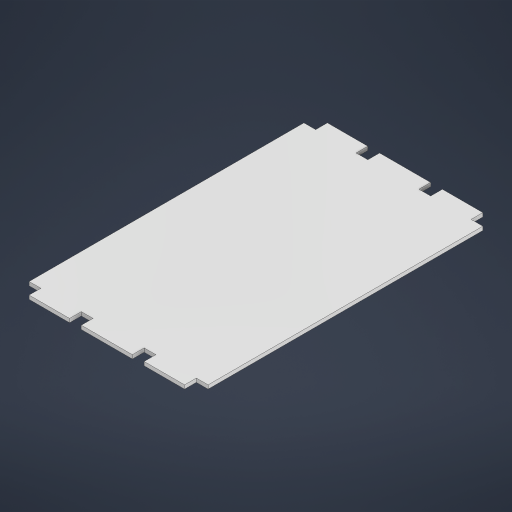
# Autodesk Inventor part: Shee
Saved by Autodesk Inventor 2024.3 (Build 283343000, 343)
## iProperties
Created: 2024-06-13
Part Number: Shee
Material: Generic
Document SubType Name: Modeling
Designer: braed
Density: 1 g/cm^3
Appearance: Default
Author: braed
Autodesk Inventor part; units mm, degrees
ref_plane "YZ Plane" through (0, 0, 0) normal (1, 0, 0) x (0, 1, 0)
ref_plane "XZ Plane" through (0, 0, 0) normal (0, 1, 0) x (-1, 0, 0)
ref_plane "XY Plane" through (0, 0, 0) normal (0, 0, 1) x (1, 0, 0)
sketch "Sketch1" plane through (0, 0, 0) normal (0, 0, 1) x (1, 0, 0)
  line L0 (0, 0) -> (304.8, 0)
  line L1 (304.8, 0) -> (304.8, 6.35)
  line L2 (304.8, 6.35) -> (0, 6.35)
  line L3 (0, 6.35) -> (0, 0)
  dimension "d0" = 304.8
  dimension "d1" = 6.35
  constraints: 8 end point, 2 parallel, 1 horizontal, 1 perpendicular
  measures "d0" distance of L2.end L1.end
  measures "d1" distance of L1.end L0.end
extrude "Extrusion1" add sketch "Sketch1" along normal blind 508
sketch "Sketch2" plane through (0, 6.35, 0) normal (0, 1, 0) x (1, 0, 0)
  line L0 (304.8, 0) -> (0, 0) construction
  line L1 (152.4, 0) -> (152.4, -508) construction
  line L2 (304.8, -508) -> (0, -508) construction
  line L3 (0, 0) -> (0, -508) construction
  line L4 (0, -254) -> (304.8, -254) construction
  line L5 (304.8, 0) -> (304.8, -508) construction
  line L6 (0, 0) -> (0, -20)
  line L7 (0, -20) -> (20, -20) construction
  line L8 (20, -20) -> (0, -20)
  line L9 (0, -20) -> (0, 0)
  line L10 (0, 0) -> (20, 0)
  line L11 (20, 0) -> (20, -20)
  line L12 (304.8, 0) -> (304.8, -20)
  line L13 (304.8, -20) -> (284.8, -20) construction
  line L14 (284.8, -20) -> (304.8, -20)
  line L15 (304.8, -20) -> (304.8, 0)
  line L16 (304.8, 0) -> (284.8, 0)
  line L17 (284.8, 0) -> (284.8, -20)
  line L18 (304.8, -508) -> (0, -508) construction
  line L19 (0, -508) -> (0, -488)
  line L20 (0, -488) -> (20, -488) construction
  line L21 (20, -488) -> (0, -488)
  line L22 (0, -488) -> (0, -508)
  line L23 (0, -508) -> (20, -508)
  line L24 (20, -508) -> (20, -488)
  line L25 (304.8, -508) -> (304.8, -488)
  line L26 (304.8, -488) -> (284.8, -488) construction
  line L27 (284.8, -488) -> (304.8, -488)
  line L28 (304.8, -488) -> (304.8, -508)
  line L29 (304.8, -508) -> (284.8, -508)
  line L30 (284.8, -508) -> (284.8, -488)
  dimension "d4" = 20
  dimension "d5" = 20
  constraints: 54 end point, 12 symmetric about line, 4 midpoint, 2 parallel, 2 perpendicular, 1 horizontal, 1 point on line
  measures "d4" distance of L0.end L6.end
  measures "d5" distance of L6.end L7.end
extrude "Extrusion2" cut sketch "Sketch2" against normal through all
sketch "Sketch3" plane through (20, 6.35, 0) normal (0, 1, 0) x (1, 0, 0)
  line L0 (0, 0) -> (264.8, 0) construction
  line L1 (132.4, 0) -> (132.4, -508) construction
  line L2 (0, -508) -> (264.8, -508) construction
  line L3 (-20, -20) -> (-20, -488) construction
  line L4 (-20, -254) -> (284.8, -254) construction
  line L5 (284.8, -20) -> (284.8, -488) construction
  line L6 (132.4, 0) -> (88.9, 0) construction
  line L7 (88.9, 0) -> (68.9, 0)
  line L8 (68.9, 0) -> (68.9, -20)
  line L9 (68.9, -20) -> (88.9, -20)
  line L10 (88.9, -20) -> (88.9, 0)
  line L11 (175.9, 0) -> (195.9, 0)
  line L12 (195.9, 0) -> (195.9, -20)
  line L13 (195.9, -20) -> (175.9, -20)
  line L14 (175.9, -20) -> (175.9, 0)
  line L15 (132.4, -508) -> (88.9, -508) construction
  line L16 (88.9, -508) -> (68.9, -508)
  line L17 (68.9, -508) -> (68.9, -488)
  line L18 (68.9, -488) -> (88.9, -488)
  line L19 (88.9, -488) -> (88.9, -508)
  line L20 (175.9, -508) -> (195.9, -508)
  line L21 (195.9, -508) -> (195.9, -488)
  line L22 (195.9, -488) -> (175.9, -488)
  line L23 (175.9, -488) -> (175.9, -508)
  point P0 (-20, 0)
  dimension "d8" = 43.5
  dimension "d9" = 20
  dimension "d10" = 20
  constraints: 40 end point, 12 symmetric about line, 4 midpoint, 2 parallel, 1 horizontal, 1 perpendicular, 1 point on line
  measures "d8" distance of L1.start L6.end
  measures "d9" distance of L9.end L8.end
  measures "d10" distance of L8.end L7.end
extrude "Extrusion3" cut sketch "Sketch3" against normal through all
body "Solid1"
